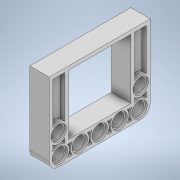
# Autodesk Inventor part: chaimber-adapter
Saved by Autodesk Inventor 2021 (Build 250183000, 183)
## iProperties
Created: 2024-03-14
Part Number: chaimber-adapter
Material: Generic
Document SubType Name: Modeling
Designer: 22hamfri
Density: 1 g/cm^3
Appearance: Default
Author: 22hamfri
Autodesk Inventor part; units mm, degrees
ref_plane "YZ Plane" through (0, 0, 0) normal (1, 0, 0) x (0, 1, 0)
ref_plane "XZ Plane" through (0, 0, 0) normal (0, 1, 0) x (-1, 0, 0)
ref_plane "XY Plane" through (0, 0, 0) normal (0, 0, 1) x (1, 0, 0)
sketch "Sketch1" plane through (0, 0, 0) normal (1, 0, 0) x (0, 1, 0)
  line L0 (0, 0) -> (0, -12.5)
  line L1 (0, -12.5) -> (25.5, -12.5)
  circle A0 centre (-3.8, 0) radius 3.8
  circle A1 centre (-3.8, 0) radius 3.1
  circle A2 centre (-3.8, 0) radius 2.575
  circle A3 centre (-3.8, -7.97) radius 3.1
  circle A4 centre (-3.8, -7.97) radius 2.575
  circle A5 centre (-3.8, -7.97) radius 3.8
  circle A6 centre (-3.8, -15.94) radius 3.1
  circle A7 centre (-3.8, -15.94) radius 2.575
  circle A8 centre (-3.8, -15.94) radius 3.8
  line L2 (25.5, -20.24) -> (25.5, -12.5)
  line L3 (-7.6, 0) -> (-7.6, -15.94)
  line L4 (-1.225, 0) -> (-6.375, 0)
  line L5 (-1.5, -3.0249) -> (-1.5, -4.9451)
  line L6 (-1.5, -10.9949) -> (-1.5, -12.9151)
  line L7 (-6.1, -4.9451) -> (-6.1, -3.0249)
  line L8 (-6.1, -12.9151) -> (-6.1, -10.9949)
  line L9 (0, 0) -> (0, 12.5)
  line L10 (0, 12.5) -> (25.5, 12.5)
  circle A9 centre (-3.8, 0) radius 3.8
  circle A10 centre (-3.8, 0) radius 3.1
  circle A11 centre (-3.8, 0) radius 2.575
  line L11 (25.5, 20.24) -> (25.5, 12.5)
  line L12 (-7.6, 0) -> (-7.6, 15.94)
  line L13 (25.5, 12.5) -> (25.5, -12.5)
  line L14 (24, 12.5) -> (24, -12.5)
  circle A12 centre (4.17, -16.44) radius 2.575
  circle A13 centre (4.17, -16.44) radius 3.1
  circle A14 centre (4.17, -16.44) radius 3.8
  line L15 (25.5, -20.24) -> (-3.8, -20.24)
  line L16 (-7.6, -16.44) -> (-7.6, -15.94)
  arc A15 (-7.6, -16.44) -> (-3.8, -20.24) centre (-3.8, -16.44) ccw
  line L17 (24, -14) -> (-0.5325, -14)
  line L18 (24, -14) -> (24, -18.74)
  line L19 (24, -18.74) -> (7.1949, -18.74)
  line L20 (1.1451, -18.74) -> (-3.8, -18.74)
  line L21 (-6.1, -16.44) -> (-6.1, -18.9649)
  arc A16 (-6.1, -16.44) -> (-3.8, -18.74) centre (-3.8, -16.44) ccw
  line L22 (4.17, -14) -> (4.17, -20.24)
  line L23 (4.92, -14) -> (4.92, -12.7147)
  line L24 (3.42, -14) -> (3.42, -12.7147)
  line L25 (25.5, 0) -> (-7.6, 0)
  line L26 (0, 0) -> (0, 12.5)
  line L27 (0, 12.5) -> (25.5, 12.5)
  circle A17 centre (-3.8, 0) radius 3.8
  circle A18 centre (-3.8, 0) radius 3.1
  circle A19 centre (-3.8, 0) radius 2.575
  circle A20 centre (-3.8, 7.97) radius 3.1
  circle A21 centre (-3.8, 7.97) radius 2.575
  circle A22 centre (-3.8, 7.97) radius 3.8
  circle A23 centre (-3.8, 15.94) radius 3.1
  circle A24 centre (-3.8, 15.94) radius 2.575
  circle A25 centre (-3.8, 15.94) radius 3.8
  line L28 (25.5, 20.24) -> (25.5, 12.5)
  line L29 (-7.6, 0) -> (-7.6, 15.94)
  line L30 (-1.5, 3.0249) -> (-1.5, 4.9451)
  line L31 (-1.5, 10.9949) -> (-1.5, 12.9151)
  line L32 (-6.1, 4.9451) -> (-6.1, 3.0249)
  line L33 (-6.1, 12.9151) -> (-6.1, 10.9949)
  circle A26 centre (-3.8, 0) radius 2.575
  circle A27 centre (-3.8, 0) radius 3.8
  circle A28 centre (-3.8, 0) radius 3.1
  line L34 (25.5, -12.5) -> (25.5, 12.5)
  line L35 (24, -12.5) -> (24, 12.5)
  circle A29 centre (4.17, 16.44) radius 2.575
  circle A30 centre (4.17, 16.44) radius 3.1
  circle A31 centre (4.17, 16.44) radius 3.8
  line L36 (25.5, 20.24) -> (-3.8, 20.24)
  line L37 (-7.6, 16.44) -> (-7.6, 15.94)
  arc A32 (-3.8, 20.24) -> (-7.6, 16.44) centre (-3.8, 16.44) ccw
  line L38 (24, 14) -> (-0.5325, 14)
  line L39 (24, 14) -> (24, 18.74)
  line L40 (24, 18.74) -> (7.1949, 18.74)
  line L41 (1.1451, 18.74) -> (-3.8, 18.74)
  line L42 (-6.1, 16.44) -> (-6.1, 18.9649)
  arc A33 (-3.8, 18.74) -> (-6.1, 16.44) centre (-3.8, 16.44) ccw
  line L43 (4.17, 14) -> (4.17, 20.24)
  line L44 (4.92, 14) -> (4.92, 12.7147)
  line L45 (3.42, 14) -> (3.42, 12.7147)
  point P0 (7.0831, 14)
  point P1 (1.2569, 14)
  point P2 (-1.231, 18.74)
  point P3 (7.0831, -14)
  point P4 (-1.231, -18.74)
  point P5 (1.2569, -14)
  dimension "d0" = 5.15
  dimension "d1" = 6.2
  dimension "d2" = 0.7
  dimension "d5" = 7.97
  dimension "d25" = 1.5
  dimension "d26" = 1.5
  dimension "d27" = 25
  dimension "d34" = 24
  dimension "d35" = 5.15
  dimension "d36" = 6.2
  dimension "d37" = 0.7
  dimension "d38" = 7.97
  dimension "d40" = 0.5
  dimension "d43" = 1.5
  dimension "d44" = 1.5
  dimension "d45" = 1.5
  dimension "d46" = 1.5
  dimension "d48" = 1.5
  dimension "d49" = 1.5
  constraints: 92 end point, 42 point on circle, 39 symmetric about line, 32 centre point, 9 point on line, 9 tangent, 8 vertical, 7 perpendicular, 5 collinear, 5 horizontal, 3 horizontal alignment, 1 equal radius, 1 line through centre, 1 midpoint, 1 parallel, 30 other
  measures "d0" diameter of A2
  measures "d1" diameter of A1
  measures "d2" radial gap between concentric circles of A1 A0
  measures "d5" distance of A1.centre A3.centre
  measures "d25" distance between parallel lines of L0 L6
  measures "d26" distance between parallel lines of L3 L8
  measures "d27" distance between parallel lines of L1 L10
  measures "d34" distance between parallel lines of L14 L0
  measures "d35" diameter of A12
  measures "d36" diameter of A13
  measures "d37" radial gap between concentric circles of A13 A14
  measures "d38" horizontal distance of A6.centre A12.centre
  measures "d40" vertical distance of A6.centre A12.centre
  measures "d43" distance between parallel lines of L15 L19
  measures "d44" distance between parallel lines of L2 L18
  measures "d45" distance between parallel lines of L17 L1
  measures "d46" distance between parallel lines of L13 L14
  measures "d48" radial gap between concentric circles of A15 A16
  measures "d49" distance between parallel lines of L23 L24
extrude "Extrusion4" add sketch "Sketch1" against normal mid plane 7.76 contours L25 A1 A0 | L0 A5 L5 A0 | A0 L30 A22 L9 | A0 L25 A1 | A5 | L0 L1 L2 L15 A14 L19 L18 L17 A8 L6 A5 | A22 L31 A25 L38 A31 L39 L40 L36 L11 L10 L9 | A22 | L25 L13 L1 L14 | L14 L10 L13 L25 | A0 L12 A22 L32 | L7 A5 L3 A0 | L8 A8 L3 A5 | A8 L20 A6 L21 | A22 L12 A25 L33 | A25 L42 A23 L41 | A8 L20 A14 L15 A15 L16 | L17 A13 L22 A14 | A14 L24 A13 L17 | L37 A32 L36 A31 L41 A25 | L38 A30 L45 A31 | A31 L43 A30 L38 | A31 L38 A30 L43 | L22 A13 L17 A14 | L21 A6 L20 A8 | A14 L23 A13 L24 | A25 L41 A23 L42 | L45 A30 L44 A31 | A14 L17 A13 L23 | L44 A30 L38 A31
extrude "Extrusion5" add sketch "Sketch1" along normal mid plane 4 contours A0 L32 A22 L30 | L5 A5 L7 A0 | L6 A8 L8 A5 | A22 L33 A25 L31 | L17 A14 L20 A8 | A25 L41 A31 L38 | L40 L39 L38 A31 | A14 L17 L18 L19
extrude "Extrusion6" add sketch "Sketch1" along normal mid plane 6.16 contours L25 A2 A1 | A1 L25 A2 | L17 A12 L22 A13 | A13 L24 A12 L17 | L38 A29 L45 A30 | A30 L43 A29 L38 | A30 L38 A29 L43 | L22 A12 L17 A13 | L21 A7 A16 L20 A6 | A6 L20 A16 A7 L21 | A13 L23 A12 L24 | L42 A24 A33 L41 A23 | A23 L41 A33 A24 L42 | L45 A29 L44 A30 | A13 L17 A12 L23 | L44 A29 L38 A30 | A3 | A20
equation "\"d25\" = d23"
equation "\"d26\" = d23"
equation "\"d20\" = d19"
equation "\"d21\" = d19"
equation "\"d22\" = d19"
equation "\"d23\" = 1.5"
equation "\"d19\" = 1.5"
body "Solid2"
